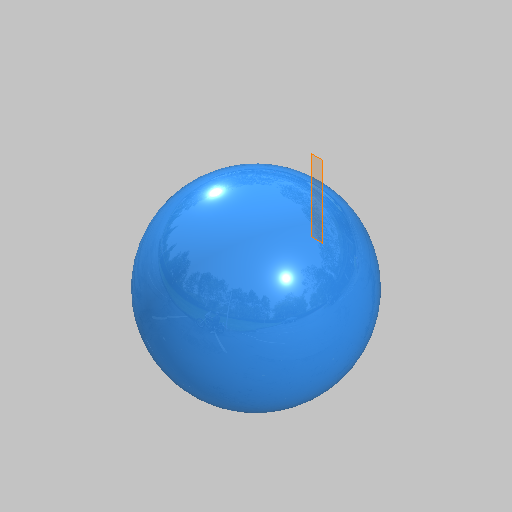
# Autodesk Inventor part: ball
Saved by Autodesk Inventor 2026 (Build 300175000, 175)
## iProperties
Created: 2026-07-30
Part Number: ball
Material: Типовые
Document SubType Name: Modeling
Designer: admin
Density: 1 g/cm^3
Appearance: Голубой
Author: admin
Autodesk Inventor part; units mm, degrees
ref_plane "YZ Plane" through (0, 0, 0) normal (1, 0, 0) x (0, 1, 0)
ref_plane "XZ Plane" through (0, 0, 0) normal (0, 1, 0) x (-1, 0, 0)
ref_plane "XY Plane" through (0, 0, 0) normal (0, 0, 1) x (1, 0, 0)
ref_plane "РабПлоскость1" through (0, 0, 0) normal (0, 0, 1) x (1, 0, 0)
sketch "Эскиз1" plane through (0, 0, 0) normal (0, 0, 1) x (1, 0, 0)
  circle A0 centre (-16.5, 0) radius 26 projected
  line L0 (-16.5, -26) -> (-16.5, 26)
  point P0 (0, 0)
  constraints: 2 end point, 2 point on circle, 1 midpoint, 1 vertical
revolve "Вращение1" add sketch "Эскиз1" angle 360 about axis through (-16.5, -26, 0) along (0, 1, 0) picked at (-24.6035, -3.0732) contours L0 A0
